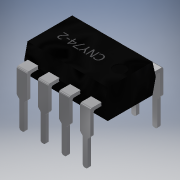
# Autodesk Inventor part: TL072
Saved by Autodesk Inventor 2018.3 (Build 223284000, 284)
## iProperties
Created: 2012-07-17
Part Number: TL072
Document SubType Name: Modeling
Designer: L.AGUERRE
Density: 8.47 g/cm^3
Description: OPTOACOPLADOR CNY74-2
Material: Genérico
Appearance: Negro
Author: laguerre
Autodesk Inventor part; units mm, degrees
ref_plane "YZ Plane" through (0, 0, 0) normal (1, 0, 0) x (0, 1, 0)
ref_plane "XZ Plane" through (0, 0, 0) normal (0, 1, 0) x (-1, 0, 0)
ref_plane "XY Plane" through (0, 0, 0) normal (0, 0, 1) x (1, 0, 0)
sketch "Boceto39" plane through (0, 0, 0) normal (0, 0, 1) x (1, 0, 0)
  line L0 (-3.1, 0) -> (-2.7, 1.75)
  line L1 (-2.7, 1.75) -> (2.7, 1.75)
  line L2 (2.7, 1.75) -> (3.1, 0)
  line L3 (3.1, 0) -> (2.7, -1.75)
  line L4 (2.7, -1.75) -> (-2.7, -1.75)
  line L5 (-2.7, -1.75) -> (-3.1, 0)
  line L6 (0, 1.75) -> (0, 1.1474) construction
  point P0 (0, 0)
  point P1 (0, -1.75)
  dimension "d373" = 5.4
  dimension "d374" = 3.5
  dimension "d375" = 6.2
  constraints: 14 end point, 3 vertical alignment, 2 horizontal alignment, 2 midpoint, 1 equal length, 1 horizontal, 1 parallel, 1 perpendicular, 2 other
  measures "d373" distance of L0.end L1.end
  measures "d374" distance between parallel lines of L1 L4
  measures "d375" distance of L2.end L0.start
extrude "Extrusión13" add sketch "Boceto39" along normal mid plane 9.7
sketch "Boceto40" plane through (-2.7, 1.75, 4.85) normal (0, 1, 0) x (1, 0, 0)
  circle A0 centre (2.7, 8.45) radius 0.75
  line L0 (0, 0) -> (5.4, 0) projected
  line L1 (5.4, 0) -> (5.4, 9.7) projected
  line L2 (5.4, 9.7) -> (0, 9.7) projected
  line L3 (0, 0) -> (0, 9.7) projected
  point P0 (2.7, 4.85)
  dimension "d378" = 1.5
  dimension "d379" = 0.5
  constraints: 1 centre point, 1 vertical alignment
  measures "d378" diameter of A0
  measures "d379" distance edge to line of A0 L2
extrude "Extrusión14" cut sketch "Boceto40" against normal blind 0.1 contours A0
sketch "Boceto41" plane through (-2.7, 1.75, 4.85) normal (0, 1, 0) x (1, 0, 0)
  line L0 (3.2517, 6.4704) -> (3.2517, 0.4631) construction
  line L1 (3.2517, 0.4631) -> (1.9852, 0.4631) construction
  line L2 (1.9852, 0.4631) -> (1.9852, 6.4704) construction
  line L3 (1.9852, 6.4704) -> (3.2517, 6.4704) construction
  spline S0 degree 2 poles (2.2128, 5.9785) (2.2128, 6.0758) (2.2784, 6.2403) (2.3441, 6.3002) knots 0 0 0 1 2 2 2
  spline S1 degree 2 poles (2.3441, 6.3002) (2.4089, 6.3602) (2.6034, 6.4258) (2.7298, 6.4258) knots 0 0 0 1 2 2 2
  spline S2 degree 2 poles (2.7298, 6.4258) (2.8554, 6.4258) (3.0418, 6.3618) (3.1107, 6.301) knots 0 0 0 1 2 2 2
  spline S3 degree 2 poles (3.1107, 6.301) (3.1779, 6.2411) (3.2484, 6.0774) (3.2484, 5.9761) knots 0 0 0 1 2 2 2
  spline S4 degree 2 poles (3.2484, 5.9761) (3.2484, 5.9258) (3.2339, 5.8375) (3.2225, 5.8002) knots 0 0 0 1 2 2 2
  spline S5 degree 2 poles (3.2225, 5.8002) (3.212, 5.7678) (3.182, 5.7006) (3.1642, 5.6673) knots 0 0 0 1 2 2 2
  line L4 (3.1642, 5.6673) -> (3.0037, 5.6673)
  line L5 (3.0037, 5.6673) -> (3.0037, 5.6779)
  spline S6 degree 2 poles (3.0037, 5.6779) (3.0199, 5.6957) (3.0653, 5.7508) (3.0872, 5.7905) knots 0 0 0 1 2 2 2
  spline S7 degree 2 poles (3.0872, 5.7905) (3.1083, 5.8286) (3.135, 5.9186) (3.135, 5.9769) knots 0 0 0 1 2 2 2
  spline S8 degree 2 poles (3.135, 5.9769) (3.135, 6.0409) (3.0823, 6.1552) (3.0321, 6.1981) knots 0 0 0 1 2 2 2
  spline S9 degree 2 poles (3.0321, 6.1981) (2.981, 6.2403) (2.8262, 6.2873) (2.7298, 6.2873) knots 0 0 0 1 2 2 2
  spline S10 degree 2 poles (2.7298, 6.2873) (2.6269, 6.2873) (2.4786, 6.2378) (2.4275, 6.1949) knots 0 0 0 1 2 2 2
  spline S11 degree 2 poles (2.4275, 6.1949) (2.3781, 6.1528) (2.3279, 6.0401) (2.3279, 5.9769) knots 0 0 0 1 2 2 2
  spline S12 degree 2 poles (2.3279, 5.9769) (2.3279, 5.9194) (2.3562, 5.8213) (2.3773, 5.7832) knots 0 0 0 1 2 2 2
  spline S13 degree 2 poles (2.3773, 5.7832) (2.3984, 5.7468) (2.4421, 5.6925) (2.4575, 5.6771) knots 0 0 0 1 2 2 2
  line L6 (2.4575, 5.6771) -> (2.4575, 5.6673)
  line L7 (2.4575, 5.6673) -> (2.2987, 5.6673)
  spline S14 degree 2 poles (2.2987, 5.6673) (2.2833, 5.7006) (2.2549, 5.7589) (2.242, 5.8002) knots 0 0 0 1 2 2 2
  spline S15 degree 2 poles (2.242, 5.8002) (2.2274, 5.844) (2.2128, 5.9186) (2.2128, 5.9785) knots 0 0 0 1 2 2 2
  line L8 (2.2306, 4.8278) -> (2.2306, 4.9769)
  line L9 (2.2306, 4.9769) -> (3.0929, 5.4194)
  line L10 (3.0929, 5.4194) -> (2.2306, 5.4194)
  line L11 (2.2306, 5.4194) -> (2.2306, 5.5434)
  line L12 (2.2306, 5.5434) -> (3.2306, 5.5434)
  line L13 (3.2306, 5.5434) -> (3.2306, 5.3545)
  line L14 (3.2306, 5.3545) -> (2.4389, 4.9518)
  line L15 (2.4389, 4.9518) -> (3.2306, 4.9518)
  line L16 (3.2306, 4.9518) -> (3.2306, 4.8278)
  line L17 (3.2306, 4.8278) -> (2.2306, 4.8278)
  line L18 (3.2306, 3.925) -> (2.6731, 4.263)
  line L19 (2.6731, 4.263) -> (2.2306, 4.263)
  line L20 (2.2306, 4.263) -> (2.2306, 4.3959)
  line L21 (2.2306, 4.3959) -> (2.6593, 4.3959)
  line L22 (2.6593, 4.3959) -> (3.2306, 4.7338)
  line L23 (3.2306, 4.7338) -> (3.2306, 4.5863)
  line L24 (3.2306, 4.5863) -> (2.7906, 4.3286)
  line L25 (2.7906, 4.3286) -> (3.2306, 4.066)
  line L26 (3.2306, 4.066) -> (3.2306, 3.925)
  line L27 (3.0807, 3.233) -> (2.2306, 3.6657)
  line L28 (2.2306, 3.6657) -> (2.2306, 3.8083)
  line L29 (2.2306, 3.8083) -> (3.1131, 3.3513)
  line L30 (3.1131, 3.3513) -> (3.1131, 3.8675)
  line L31 (3.1131, 3.8675) -> (3.2306, 3.8675)
  line L32 (3.2306, 3.8675) -> (3.2306, 3.233)
  line L33 (3.2306, 3.233) -> (3.0807, 3.233)
  line L34 (2.5742, 2.4672) -> (2.5742, 2.5863)
  line L35 (2.5742, 2.5863) -> (2.2306, 2.5863)
  line L36 (2.2306, 2.5863) -> (2.2306, 2.7151)
  line L37 (2.2306, 2.7151) -> (2.5742, 2.7151)
  line L38 (2.5742, 2.7151) -> (2.5742, 3.1568)
  line L39 (2.5742, 3.1568) -> (2.7152, 3.1568)
  line L40 (2.7152, 3.1568) -> (3.2306, 2.7095)
  line L41 (3.2306, 2.7095) -> (3.2306, 2.5863)
  line L42 (3.2306, 2.5863) -> (2.682, 2.5863)
  line L43 (2.682, 2.5863) -> (2.682, 2.4672)
  line L44 (2.682, 2.4672) -> (2.5742, 2.4672)
  line L45 (2.682, 2.7151) -> (3.0726, 2.7151)
  line L46 (3.0726, 2.7151) -> (2.682, 3.0515)
  line L47 (2.682, 3.0515) -> (2.682, 2.7151)
  line L48 (2.6074, 1.9939) -> (2.6074, 2.3724)
  line L49 (2.6074, 2.3724) -> (2.729, 2.3724)
  line L50 (2.729, 2.3724) -> (2.729, 1.9939)
  line L51 (2.729, 1.9939) -> (2.6074, 1.9939)
  line L52 (2.2306, 1.2443) -> (2.2306, 1.861)
  line L53 (2.2306, 1.861) -> (2.3724, 1.861)
  spline S16 degree 2 poles (2.3724, 1.861) (2.4348, 1.7946) (2.5507, 1.6763) (2.6131, 1.6195) knots 0 0 0 1 2 2 2
  spline S17 degree 2 poles (2.6131, 1.6195) (2.7387, 1.5053) (2.8894, 1.4218) (2.9697, 1.4218) knots 0 0 0 1 2 2 2
  spline S18 degree 2 poles (2.9697, 1.4218) (3.0118, 1.4218) (3.075, 1.4477) (3.0953, 1.4712) knots 0 0 0 1 2 2 2
  spline S19 degree 2 poles (3.0953, 1.4712) (3.1155, 1.4947) (3.1358, 1.5563) (3.1358, 1.5936) knots 0 0 0 1 2 2 2
  spline S20 degree 2 poles (3.1358, 1.5936) (3.1358, 1.6293) (3.118, 1.7022) (3.1042, 1.7354) knots 0 0 0 1 2 2 2
  spline S21 degree 2 poles (3.1042, 1.7354) (3.0929, 1.7638) (3.0604, 1.8164) (3.0491, 1.8327) knots 0 0 0 1 2 2 2
  line L54 (3.0491, 1.8327) -> (3.0491, 1.8399)
  line L55 (3.0491, 1.8399) -> (3.1917, 1.8399)
  spline S22 degree 2 poles (3.1917, 1.8399) (3.212, 1.7986) (3.2517, 1.6503) (3.2517, 1.5839) knots 0 0 0 1 2 2 2
  spline S23 degree 2 poles (3.2517, 1.5839) (3.2517, 1.4437) (3.1034, 1.2857) (2.977, 1.2857) knots 0 0 0 1 2 2 2
  spline S24 degree 2 poles (2.977, 1.2857) (2.9178, 1.2857) (2.8189, 1.3132) (2.7768, 1.3375) knots 0 0 0 1 2 2 2
  spline S25 degree 2 poles (2.7768, 1.3375) (2.733, 1.3618) (2.6471, 1.4323) (2.6058, 1.4712) knots 0 0 0 1 2 2 2
  spline S26 degree 2 poles (2.6058, 1.4712) (2.5369, 1.5344) (2.3894, 1.6892) (2.3465, 1.7354) knots 0 0 0 1 2 2 2
  line L56 (2.3465, 1.7354) -> (2.3465, 1.2443)
  line L57 (2.3465, 1.2443) -> (2.2306, 1.2443)
  point P0 (2.7, 4.85)
  constraints: 2 other
emboss "Repujado1" sketch "Boceto41" operation cut depth 0.01 direction (0, -1, 0)
sketch "Boceto42" plane through (0, 0, 0) normal (1, 0, 0) x (0, 1, 0)
  line L0 (0.2, 4.45) -> (-0.2, 4.45)
  line L1 (-0.2, 4.45) -> (-0.2, 3.2)
  line L2 (-0.2, 3.2) -> (0.2, 3.2)
  line L3 (0.2, 3.2) -> (0.2, 4.45)
  line L4 (0.2, 1.9) -> (-0.2, 1.9)
  line L5 (-0.2, 1.9) -> (-0.2, 0.65)
  line L6 (-0.2, 0.65) -> (0.2, 0.65)
  line L7 (0.2, 0.65) -> (0.2, 1.9)
  line L8 (0.2, -0.65) -> (-0.2, -0.65)
  line L9 (-0.2, -0.65) -> (-0.2, -1.9)
  line L10 (-0.2, -1.9) -> (0.2, -1.9)
  line L11 (0.2, -1.9) -> (0.2, -0.65)
  line L12 (0.2, -3.2) -> (-0.2, -3.2)
  line L13 (-0.2, -3.2) -> (-0.2, -4.45)
  line L14 (-0.2, -4.45) -> (0.2, -4.45)
  line L15 (0.2, -4.45) -> (0.2, -3.2)
  point P0 (0, 0)
  point P1 (0, 0.65)
  point P2 (0, -0.65)
  point P3 (0, -3.2)
  point P4 (0, -1.9)
  point P5 (0, 3.2)
  point P6 (0, 1.9)
  dimension "d384" = 1.25
  dimension "d385" = 0.4
  dimension "d386" = 1.3
  dimension "d387" = 1.3
  dimension "d388" = 1.3
  dimension "d389" = 0.65
  constraints: 32 end point, 8 parallel, 6 equal length, 6 midpoint, 4 horizontal, 4 perpendicular, 4 vertical alignment
  measures "d384" distance of L0.end L1.end
  measures "d385" distance of L0.start L0.end
  measures "d386" distance between parallel lines of L8 L6
  measures "d387" distance between parallel lines of L4 L2
  measures "d388" distance from line of L12 L10.end
  measures "d389" distance of point (0, 0) point (0, 0.65)
extrude "Extrusión15" add sketch "Boceto42" along normal mid plane 8
sketch "Boceto43" plane through (4, 0, 0) normal (1, 0, 0) x (0, 0, -1)
  line L0 (-4.45, 0.2) -> (-3.2, 0.2) projected
  line L1 (-4.45, -0.2) -> (-4.45, 0.2) projected
  line L2 (-3.2, -0.2) -> (-4.45, -0.2) projected
  line L3 (-3.2, 0.2) -> (-3.2, -0.2) projected
  line L4 (-1.9, 0.2) -> (-0.65, 0.2) projected
  line L5 (-1.9, -0.2) -> (-1.9, 0.2) projected
  line L6 (-0.65, -0.2) -> (-1.9, -0.2) projected
  line L7 (-0.65, 0.2) -> (-0.65, -0.2) projected
  line L8 (0.65, 0.2) -> (1.9, 0.2) projected
  line L9 (0.65, -0.2) -> (0.65, 0.2) projected
  line L10 (1.9, -0.2) -> (0.65, -0.2) projected
  line L11 (1.9, 0.2) -> (1.9, -0.2) projected
  line L12 (3.2, 0.2) -> (4.45, 0.2) projected
  line L13 (3.2, -0.2) -> (3.2, 0.2) projected
  line L14 (4.45, -0.2) -> (3.2, -0.2) projected
  line L15 (4.45, 0.2) -> (4.45, -0.2) projected
  line L16 (-4.45, 0.2) -> (-3.2, 0.2)
  line L17 (-3.2, 0.2) -> (-3.2, -2.775)
  line L18 (-4.45, -2.775) -> (-4.45, 0.2)
  line L19 (-3.2, -2.775) -> (-3.525, -3.1)
  line L20 (-3.525, -3.1) -> (-3.525, -6.3)
  line L21 (-3.525, -6.3) -> (-4.125, -6.3)
  line L22 (-4.125, -6.3) -> (-4.125, -3.1)
  line L23 (-4.125, -3.1) -> (-4.45, -2.775)
  line L24 (-1.9, 0.2) -> (-0.65, 0.2)
  line L25 (-0.65, 0.2) -> (-0.65, -2.775)
  line L26 (-1.9, -2.775) -> (-1.9, 0.2)
  line L27 (0.65, 0.2) -> (1.9, 0.2)
  line L28 (1.9, 0.2) -> (1.9, -2.775)
  line L29 (0.65, -2.775) -> (0.65, 0.2)
  line L30 (3.2, 0.2) -> (4.45, 0.2)
  line L31 (4.45, 0.2) -> (4.45, -2.775)
  line L32 (3.2, -2.775) -> (3.2, 0.2)
  line L33 (-0.65, -2.775) -> (-0.975, -3.1)
  line L34 (-0.975, -3.1) -> (-0.975, -6.3)
  line L35 (-0.975, -6.3) -> (-1.575, -6.3)
  line L36 (-1.575, -6.3) -> (-1.575, -3.1)
  line L37 (-1.575, -3.1) -> (-1.9, -2.775)
  line L38 (0.65, -2.775) -> (0.975, -3.1)
  line L39 (0.975, -3.1) -> (0.975, -6.3)
  line L40 (0.975, -6.3) -> (1.575, -6.3)
  line L41 (1.575, -6.3) -> (1.575, -3.1)
  line L42 (1.575, -3.1) -> (1.9, -2.775)
  line L43 (3.2, -2.775) -> (3.525, -3.1)
  line L44 (3.525, -3.1) -> (3.525, -6.3)
  line L45 (3.525, -6.3) -> (4.125, -6.3)
  line L46 (4.125, -6.3) -> (4.125, -3.1)
  line L47 (4.125, -3.1) -> (4.45, -2.775)
  point P0 (0, 0)
  point P1 (-3.825, -6.3)
  point P2 (-3.825, 0.2)
  point P3 (-1.275, -6.3)
  point P4 (-1.275, 0.2)
  point P5 (1.275, -6.3)
  point P6 (1.275, 0.2)
  point P7 (3.825, -6.3)
  point P8 (3.825, 0.2)
  dimension "d392" = 0.6
  dimension "d393" = 6.5
  dimension "d394" = 3.3
  constraints: 64 end point, 17 perpendicular, 10 horizontal alignment, 8 midpoint, 8 parallel, 6 equal length, 4 horizontal, 4 vertical alignment
  measures "d392" distance between parallel lines of L20 L22
  measures "d393" distance between parallel lines of L12 L45
  measures "d394" distance from line of L0 L22.end
extrude "Extrusión16" add sketch "Boceto43" along normal blind 0.4
sketch "Boceto44" plane through (-4, 0, 0) normal (-1, 0, 0) x (0, 0, 1)
  line L0 (-3.2, -0.2) -> (-4.45, -0.2) projected
  line L1 (-3.2, 0.2) -> (-3.2, -0.2) projected
  line L2 (-4.45, 0.2) -> (-3.2, 0.2) projected
  line L3 (-4.45, -0.2) -> (-4.45, 0.2) projected
  line L4 (-0.65, -0.2) -> (-1.9, -0.2) projected
  line L5 (-0.65, 0.2) -> (-0.65, -0.2) projected
  line L6 (-1.9, 0.2) -> (-0.65, 0.2) projected
  line L7 (-1.9, -0.2) -> (-1.9, 0.2) projected
  line L8 (1.9, -0.2) -> (0.65, -0.2) projected
  line L9 (1.9, 0.2) -> (1.9, -0.2) projected
  line L10 (0.65, 0.2) -> (1.9, 0.2) projected
  line L11 (0.65, -0.2) -> (0.65, 0.2) projected
  line L12 (4.45, -0.2) -> (3.2, -0.2) projected
  line L13 (4.45, 0.2) -> (4.45, -0.2) projected
  line L14 (3.2, 0.2) -> (4.45, 0.2) projected
  line L15 (3.2, -0.2) -> (3.2, 0.2) projected
  line L16 (3.2, -0.2) -> (4.45, -0.2) projected
  line L17 (3.2, -2.775) -> (3.2, -0.2) projected
  line L18 (3.525, -3.1) -> (3.2, -2.775) projected
  line L19 (3.525, -6.3) -> (3.525, -3.1) projected
  line L20 (4.125, -6.3) -> (3.525, -6.3) projected
  line L21 (4.125, -3.1) -> (4.125, -6.3) projected
  line L22 (4.45, -2.775) -> (4.125, -3.1) projected
  line L23 (4.45, -0.2) -> (4.45, -2.775) projected
  line L24 (0.65, -0.2) -> (1.9, -0.2) projected
  line L25 (0.65, -2.775) -> (0.65, -0.2) projected
  line L26 (0.975, -3.1) -> (0.65, -2.775) projected
  line L27 (0.975, -6.3) -> (0.975, -3.1) projected
  line L28 (1.575, -6.3) -> (0.975, -6.3) projected
  line L29 (1.575, -3.1) -> (1.575, -6.3) projected
  line L30 (1.9, -2.775) -> (1.575, -3.1) projected
  line L31 (1.9, -0.2) -> (1.9, -2.775) projected
  line L32 (-1.9, -0.2) -> (-0.65, -0.2) projected
  line L33 (-1.9, -2.775) -> (-1.9, -0.2) projected
  line L34 (-1.575, -3.1) -> (-1.9, -2.775) projected
  line L35 (-1.575, -6.3) -> (-1.575, -3.1) projected
  line L36 (-0.975, -6.3) -> (-1.575, -6.3) projected
  line L37 (-0.975, -3.1) -> (-0.975, -6.3) projected
  line L38 (-0.65, -2.775) -> (-0.975, -3.1) projected
  line L39 (-0.65, -0.2) -> (-0.65, -2.775) projected
  line L40 (-4.45, -0.2) -> (-3.2, -0.2) projected
  line L41 (-4.45, -2.775) -> (-4.45, -0.2) projected
  line L42 (-4.125, -3.1) -> (-4.45, -2.775) projected
  line L43 (-4.125, -6.3) -> (-4.125, -3.1) projected
  line L44 (-3.525, -6.3) -> (-4.125, -6.3) projected
  line L45 (-3.525, -3.1) -> (-3.525, -6.3) projected
  line L46 (-3.2, -2.775) -> (-3.525, -3.1) projected
  line L47 (-3.2, -0.2) -> (-3.2, -2.775) projected
  point P0 (0, 0)
extrude "Extrusión17" add sketch "Boceto44" along normal blind 0.4
fillet "Empalme44" radius 0.2 64 edges at (4.2, -6.3, 3.525) (4.2, -6.3, 4.125) (4.2, -3.1, 3.525) (4.2, -2.775, 3.2) (4.2, -3.1, 0.975) (4.2, -2.775, 0.65) (4.2, -6.3, 0.975) (4.2, -6.3, 1.575) (4.2, -6.3, -1.575) (4.2, -6.3, -0.975) (-4.2, -6.3, 4.125) (-4.2, -6.3, 3.525) (4.2, -6.3, -4.125) (-4.2, -6.3, 0.975) (-4.2, -6.3, 1.575) (4.2, -6.3, -3.525) (-4.2, -3.1, 3.525) (-4.2, -2.775, 3.2) (-4.2, -3.1, 0.975) (-4.2, -2.775, 0.65) (-4.2, -3.1, -1.575) (-4.2, -2.775, -1.9) (-4.2, -3.1, -4.125) (-4.2, -2.775, -4.45) (-4.2, -6.3, -4.125) (-4.2, -6.3, -3.525) (-4.2, -6.3, -1.575) (-4.2, -6.3, -0.975) (4.2, -3.1, -1.575) (4.2, -2.775, -1.9) (4.2, -3.1, -4.125) (4.2, -2.775, -4.45) (4.2, -3.1, -3.525) (4.2, -2.775, -3.2) (4.2, -3.1, -0.975) (4.2, -2.775, -0.65) (4.2, -3.1, 1.575) (4.2, -2.775, 1.9) (4.2, -3.1, 4.125) (4.2, -2.775, 4.45) (-4.2, -3.1, -3.525) (-4.2, -2.775, -3.2) (-4.2, -3.1, -0.975) (-4.2, -2.775, -0.65) (-4.2, -3.1, 1.575) (-4.2, -2.775, 1.9) (-4.2, -3.1, 4.125) (-4.2, -2.775, 4.45) (4.4, 0.2, 3.825) (4.4, 0.2, 1.275) (4.4, 0.2, -1.275) (4.4, 0.2, -3.825) (-4.4, 0.2, 3.825) (-4.4, 0.2, 1.275) (-4.4, 0.2, -1.275) (-4.4, 0.2, -3.825) (-4, -0.2, 3.825) (-4, -0.2, 1.275) (-4, -0.2, -1.275) (-4, -0.2, -3.825) (4, -0.2, -3.825) (4, -0.2, -1.275) (4, -0.2, 1.275) (4, -0.2, 3.825)
